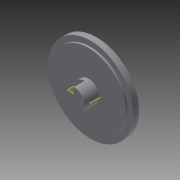
# Autodesk Inventor part: Caps 8mm Square Rounded Caps Male2
Saved by Autodesk Inventor 2018 (Build 220112000, 112)
## iProperties
Created: 2017-12-12
Part Number: Caps 8mm Square Rounded Caps Male2
Material: Generic
Document SubType Name: Modeling
Designer: Rus
Density: 1 g/cm^3
Appearance: Default
Author: Rus
Autodesk Inventor part; units mm, degrees
ref_plane "YZ Plane" through (0, 0, 0) normal (1, 0, 0) x (0, 1, 0)
ref_plane "XZ Plane" through (0, 0, 0) normal (0, 1, 0) x (-1, 0, 0)
ref_plane "XY Plane" through (0, 0, 0) normal (0, 0, 1) x (1, 0, 0)
sketch "Sketch1" plane through (0, 0, 0) normal (0, 1, 0) x (-1, 0, 0)
  circle A0 centre (0, 0) radius 4
  line L0 (0, 0) -> (4, 0) construction
  line L1 (0, 0) -> (0, -4) construction
  line L2 (0, 0) -> (-4, 0) construction
  line L3 (0, 0) -> (0, 4) construction
  dimension "d0" = 8
  constraints: 8 end point, 4 point on circle, 2 point on line, 1 centre point, 1 coincident, 1 horizontal, 1 perpendicular
  measures "d0" diameter of A0
extrude "Extrusion1" add sketch "Sketch1" against normal blind 3.5
ref_plane "Work Plane1" through (0, 0, 0) normal (0, 0, 1) x (1, 0, 0)
sketch "Sketch2" plane through (0, 0, 0) normal (0, 0, 1) x (1, 0, 0)
  line L0 (-4, 0) -> (4, 0) projected
  line L1 (4, 0) -> (14, 0)
  line L2 (16, 0.75) -> (16, 3)
  line L3 (14.5, 3.75) -> (12.5, 3.75)
  line L4 (0, 0) -> (0, 1.25)
  line L5 (4, 0) -> (4, 1.5959) construction
  line L6 (16, 0.75) -> (14, 0.75)
  line L7 (14, 0.75) -> (14, 0)
  line L8 (16, 3) -> (14.5, 3.75)
  line L9 (12.5, 2.5) -> (12.5, 3.75)
  line L10 (5.8632, 1.8363) -> (6, 1.7244)
  line L11 (6, 1.7244) -> (6.1119, 1.8612)
  line L12 (4.1119, 1.6612) -> (4, 1.5244)
  line L13 (4, 1.5244) -> (3.8632, 1.6363)
  line L14 (1.8632, 1.4363) -> (2, 1.3244)
  line L15 (2, 1.3244) -> (2.1119, 1.4612)
  line L16 (0, 1.25) -> (1.8632, 1.4363)
  line L17 (2.1119, 1.4612) -> (3.8632, 1.6363)
  line L18 (4.1119, 1.6612) -> (5.8632, 1.8363)
  line L19 (4, 1.5244) -> (4, 3.125) construction
  line L20 (6, 1.7244) -> (6, 3.125) construction
  line L21 (6, 3.125) -> (4, 3.125) construction
  line L22 (4, 3.125) -> (2, 3.125) construction
  line L23 (2, 3.125) -> (0, 3.125) construction
  line L24 (1.8632, 1.4363) -> (2.1119, 1.4612) construction
  line L25 (3.8632, 1.6363) -> (4.1119, 1.6612) construction
  line L26 (5.8632, 1.8363) -> (6.1119, 1.8612) construction
  line L27 (1.9876, 1.4488) -> (2, 1.3244) construction
  line L28 (4, 1.65) -> (4, 1.5244) construction
  line L29 (2, 1.3244) -> (2, 3.125) construction
  line L30 (7.8632, 2.0363) -> (8, 1.9244)
  line L31 (8, 1.9244) -> (8.1119, 2.0612)
  line L32 (8, 1.9244) -> (8, 3.125) construction
  line L33 (6.1119, 1.8612) -> (7.8632, 2.0363)
  line L34 (8.1119, 2.0612) -> (12.5, 2.5)
  line L35 (8, 3.125) -> (6, 3.125) construction
  line L36 (8, 3.125) -> (12.5, 3.125) construction
  point P0 (6, 1.85)
  dimension "d8" = 16
  dimension "d11" = 14
  dimension "d12" = 0.75
  dimension "d13" = 3
  dimension "d14" = 0.75
  dimension "d15" = 1.5
  dimension "d16" = 1.25
  dimension "d19" = 3.5
  dimension "d23" = 1.25
  dimension "d25" = 0.125
  dimension "d26" = 2
  dimension "d32" = 2
  constraints: 72 end point, 13 collinear, 11 perpendicular, 9 equal length, 6 point on line, 6 vertical, 3 horizontal, 2 midpoint
  measures "d8" distance between parallel lines of L2 L4
  measures "d11" distance between parallel lines of L7 L4
  measures "d12" distance of L6.end L1.end
  measures "d13" distance between parallel lines of L3 L6
  measures "d14" distance from line of L2.end L3
  measures "d15" distance from line of L2 L3.start
  measures "d16" distance of L4.start L4.end
  measures "d19" horizontal distance of L3.end L2.end
  measures "d23" vertical distance of L4.end L9.start
  measures "d25" distance of L27.start L14.end
  measures "d26" distance of L19.end L22.end
  measures "d32" distance of L22.end L23.end
revolve "Revolution1" add sketch "Sketch2" angle 360 about axis through (0, 0, 0) along (0, 1, 0)
sketch "Sketch3" plane through (0, -3.5, 0) normal (0, -1, 0) x (1, 0, 0)
  point P0 (0, 0)
  point P1 (0, 0)
  constraints: 1 coincident
sketch "Sketch4" plane through (0, -3.5, 0) normal (0, -1, 0) x (1, 0, 0)
  circle A0 centre (0, 0) radius 4 projected
  circle A1 centre (0, 0) radius 4 projected
  arc A2 (0, -4) -> (0, 4) centre (0, 0) ccw
  line L0 (0, 4) -> (0, -4)
  constraints: 2 end point, 2 point on circle, 2 vertical, 2 vertical alignment, 1 centre point, 1 coincident, 2 other
extrude "Extrusion2" add sketch "Sketch4" along normal blind 2 contours A0 L0 picked at (0.5785, 1.2013)
sketch "Sketch5" plane through (0, -3.5, 0) normal (0, -1, 0) x (1, 0, 0)
  line L0 (0, -4) -> (0, 4) projected
  arc A0 (0, 4) -> (0, -4) centre (0, 0) ccw projected
extrude "Extrusion3" cut sketch "Sketch5" against normal blind 2
body "Solid1"
